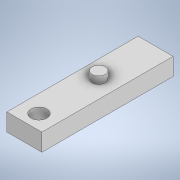
# Autodesk Inventor part: limit_switch_upper_mount
Saved by Autodesk Inventor 2022 (Build 260153000, 153)
## iProperties
Created: 2022-02-08
Part Number: limit_switch_upper_mount
Material: Generic
Document SubType Name: Modeling
Designer: kylem
Density: 1 g/cm^3
Appearance: Default
Author: kylem
Autodesk Inventor part; units mm, degrees
ref_plane "YZ Plane" through (0, 0, 0) normal (1, 0, 0) x (0, 1, 0)
ref_plane "XZ Plane" through (0, 0, 0) normal (0, 1, 0) x (-1, 0, 0)
ref_plane "XY Plane" through (0, 0, 0) normal (0, 0, 1) x (1, 0, 0)
sketch "Sketch1" plane through (0, 0, 0) normal (0, 1, 0) x (-1, 0, 0)
  line L0 (0, 0) -> (12, 0)
  line L1 (12, 0) -> (12, -45)
  line L2 (12, -45) -> (0, -45)
  line L3 (0, -45) -> (0, 0)
  dimension "d0" = 12
  dimension "d1" = 45
  constraints: 8 end point, 2 parallel, 1 horizontal, 1 perpendicular
  measures "d0" distance of L1.end L2.end
  measures "d1" distance of L0.end L1.end
extrude "Extrusion1" add sketch "Sketch1" along normal blind 6
sketch "Sketch2" plane through (0, 6, 0) normal (0, 1, 0) x (1, 0, 0)
  line L0 (-12, 0) -> (0, 0) projected
  line L1 (-6, 0) -> (-6, 5)
  circle A0 centre (-6, 5) radius 2.75
  dimension "d4" = 5
  dimension "d5" = 5.5
  constraints: 2 end point, 1 centre point, 1 coincident, 1 midpoint, 1 vertical
  measures "d4" distance of L1.start L1.end
  measures "d5" diameter of A0
extrude "Extrusion2" cut sketch "Sketch2" against normal blind 6
sketch "Sketch3" plane through (0, 6, 0) normal (0, 1, 0) x (1, 0, 0)
  circle A0 centre (-6, 5) radius 2.75 projected
  line L0 (-6, 5) -> (-6, 25.5)
  circle A1 centre (-6, 25.5) radius 2.25
  point P0 (0, 0)
  dimension "d8" = 20.5
  dimension "d9" = 4.5
  constraints: 2 end point, 1 centre point, 1 coincident, 1 vertical
  measures "d8" distance of L0.start L0.end
  measures "d9" diameter of A1
extrude "Extrusion3" add sketch "Sketch3" along normal blind 2.5 contours A1
body "Solid1"
